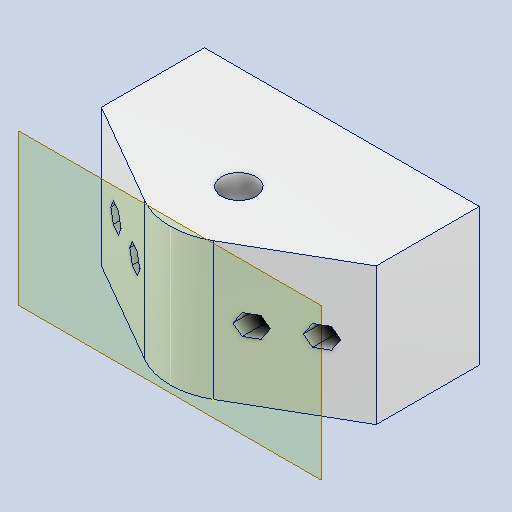
# Autodesk Inventor part: encatre sin fin
Saved by Autodesk Inventor 2023 (Build 270158000, 158)
## iProperties
Created: 2023-04-13
Part Number: encatre sin fin
Material: Aluminum 6061
Document SubType Name: Modeling
Designer: sebas
Density: 2.7 g/cm^3
Appearance: Aluminum - Flat
Author: sebas
Autodesk Inventor part; units mm, degrees
ref_plane "YZ Plane" through (0, 0, 0) normal (1, 0, 0) x (0, 1, 0)
ref_plane "XZ Plane" through (0, 0, 0) normal (0, 1, 0) x (-1, 0, 0)
ref_plane "XY Plane" through (0, 0, 0) normal (0, 0, 1) x (1, 0, 0)
sketch "Sketch1" plane through (0, 0, 0) normal (0, 1, 0) x (-1, 0, 0)
  circle A0 centre (0, 0) radius 20
  line L0 (8, 0) -> (4, -6.9282)
  line L1 (4, -6.9282) -> (-4, -6.9282)
  line L2 (-4, -6.9282) -> (-8, 0)
  line L3 (-8, 0) -> (-4, 6.9282)
  line L4 (-4, 6.9282) -> (4, 6.9282)
  line L5 (4, 6.9282) -> (8, 0)
  dimension "d1" = 40
  dimension "d5" = 8
  constraints: 12 end point, 2 coincident, 1 centre point, 13 other
  measures "d1" diameter of A0
  measures "d5" distance of A0.centre L0.start
extrude "Extrusion1" add sketch "Sketch1" along normal blind 40
sketch "Sketch2" plane through (0, 40, 0) normal (0, 1, 0) x (1, 0, 0)
  line L0 (-8, 0) -> (-4, 6.9282) projected
  line L1 (-8, 0) -> (-4, 6.9282)
  line L2 (-4, 6.9282) -> (4, 6.9282)
  line L3 (4, 6.9282) -> (8, 0)
  line L4 (8, 0) -> (4, -6.9282)
  line L5 (4, -6.9282) -> (-4, -6.9282)
  line L6 (-4, -6.9282) -> (-8, 0)
  point P0 (0, 0)
  point P1 (0, 0)
  constraints: 12 end point, 1 coincident, 13 other
extrude "Extrusion2" add sketch "Sketch2" against normal blind 10
sketch "Sketch3" plane through (0, 40, 0) normal (0, 1, 0) x (1, 0, 0)
  circle A0 centre (0, 0) radius 5
  dimension "d8" = 10
  constraints: 1 centre point, 1 coincident
  measures "d8" diameter of A0
extrude "Extrusion3" cut sketch "Sketch3" against normal blind 10
sketch "Sketch4" plane through (0, 40, 0) normal (0, 1, 0) x (1, 0, 0)
  circle A0 centre (0, 0) radius 20 projected
  line L0 (20, 0) -> (40, 0)
  line L1 (40, 0) -> (40, 20)
  line L2 (40, 20) -> (0, 20)
  line L3 (-20, 20) -> (-40, 20)
  line L4 (-40, 20) -> (-40, 0)
  line L5 (-40, 0) -> (-20, 0)
  line L6 (-20, 20) -> (0, 20)
  line L7 (-40, 0) -> (-10, -17.3205)
  line L8 (40, 0) -> (10, -17.3205)
  circle A1 centre (0, 0) radius 20
  circle A2 centre (0, 0) radius 20
  dimension "d11" = 20
  dimension "d12" = 20
  constraints: 18 end point, 5 point on circle, 4 point on line, 4 tangent, 2 centre point, 2 coincident, 2 concentric, 2 perpendicular, 1 collinear, 1 horizontal
  measures "d11" distance of L0.start L0.end
  measures "d12" distance of L3.start L3.end
extrude "Extrusion4" add sketch "Sketch4" against normal blind 40 contours L0 L8 A0 | A0 L2 L1 L0 | A0 L5 L4 L3 L6 | A0 L7 L5
sketch "Sketch5" plane through (40, 40, -20) normal (0, 0, -1) x (-1, 0, 0)
  line L0 (0, 0) -> (0, -40) projected
  line L1 (0, -20) -> (80, -20)
  line L2 (80, 0) -> (80, -40) projected
  line L3 (0, -20) -> (10, -20)
  circle A0 centre (10, -20) radius 3
  line L4 (13, -20) -> (23, -20)
  circle A1 centre (23, -20) radius 3
  line L5 (40, -40) -> (40, 0)
  circle A2 centre (70, -20) radius 3
  circle A3 centre (57, -20) radius 3
  dimension "d16" = 6
  dimension "d15" = 10
  dimension "d17" = 10
  dimension "d18" = 6
  constraints: 8 end point, 3 centre point, 2 coincident, 2 midpoint, 2 point on line, 2 symmetric about line, 1 horizontal alignment, 1 vertical, 4 other
  measures "d15" distance of L1.start L3.end
  measures "d17" distance of L4.start L4.end
  measures "d18" diameter of A1
extrude "Extrusion5" cut sketch "Sketch5" along normal mid plane 80
sketch "Sketch6" plane through (0, 40, 0) normal (0, 1, 0) x (1, 0, 0)
  line L0 (-40, 20) -> (-40, 15)
  line L1 (-40, 0) -> (-40, 20) projected
  line L2 (-40, 15) -> (44.9562, 15)
  line L3 (44.9562, 15) -> (44.9562, 24.7883)
  line L4 (44.9562, 24.7883) -> (-40, 24.7883)
  line L5 (-40, 24.7883) -> (-40, 20)
  point P0 (0, 0)
  dimension "d21" = 5
  constraints: 10 end point, 4 perpendicular, 2 point on line
  measures "d21" distance of L0.start L0.end
extrude "Extrusion6" cut sketch "Sketch6" against normal through all
sketch "Sketch7" plane through (10, 0, 17.3205) normal (0.5, 0, 0.8660254) x (0.8660254, 0, -0.5)
  point P0 (0, 0)
ref_plane "Work Plane1" through (0, 0, 20) normal (0, 0, -1) x (-1, 0, 0)
sketch "Sketch8" plane through (0, 0, 20) normal (0, 0, -1) x (-1, 0, 0)
  circle A0 centre (-30, 20) radius 3 projected
  line L0 (-28.2679, 23) -> (-26.5359, 20)
  line L1 (-26.5359, 20) -> (-28.2679, 17)
  line L2 (-28.2679, 17) -> (-31.7321, 17)
  line L3 (-31.7321, 17) -> (-33.4641, 20)
  line L4 (-33.4641, 20) -> (-31.7321, 23)
  line L5 (-31.7321, 23) -> (-28.2679, 23)
  circle A1 centre (-17, 20) radius 3 projected
  line L6 (-15.2679, 23) -> (-13.5359, 20)
  line L7 (-13.5359, 20) -> (-15.2679, 17)
  line L8 (-15.2679, 17) -> (-18.7321, 17)
  line L9 (-18.7321, 17) -> (-20.4641, 20)
  line L10 (-20.4641, 20) -> (-18.7321, 23)
  line L11 (-18.7321, 23) -> (-15.2679, 23)
  circle A2 centre (17, 20) radius 3 projected
  line L12 (18.7321, 23) -> (20.4641, 20)
  line L13 (20.4641, 20) -> (18.7321, 17)
  line L14 (18.7321, 17) -> (15.2679, 17)
  line L15 (15.2679, 17) -> (13.5359, 20)
  line L16 (13.5359, 20) -> (15.2679, 23)
  line L17 (15.2679, 23) -> (18.7321, 23)
  circle A3 centre (30, 20) radius 3 projected
  line L18 (31.7321, 23) -> (33.4641, 20)
  line L19 (33.4641, 20) -> (31.7321, 17)
  line L20 (31.7321, 17) -> (28.2679, 17)
  line L21 (28.2679, 17) -> (26.5359, 20)
  line L22 (26.5359, 20) -> (28.2679, 23)
  line L23 (28.2679, 23) -> (31.7321, 23)
  point P0 (0, 0)
  point P1 (-30, 23)
  point P2 (-17, 23)
  point P3 (17, 23)
  point P4 (30, 23)
  constraints: 48 end point, 4 coincident, 4 midpoint, 4 vertical alignment, 3 point on line, 56 other
extrude "Extrusion7" cut sketch "Sketch8" along normal blind 25
sketch "Sketch9" plane through (0, 40, 0) normal (0, 1, 0) x (1, 0, 0)
  line L0 (40, 15) -> (-40, 15) projected
  line L1 (-40, 15) -> (-40, 30)
  line L2 (-40, 0) -> (-40, 15) projected
  line L3 (-40, 30) -> (40, 30)
  line L4 (40, 15) -> (40, 0) projected
  line L5 (40, 30) -> (40, 15)
  line L6 (40, 15) -> (-40, 15)
  point P0 (0, 0)
  dimension "d26" = 15
  constraints: 8 end point, 2 collinear, 2 perpendicular
  measures "d26" distance of L0.end L1.end
extrude "Extrusion8" add sketch "Sketch9" against normal blind 40
body "Solid1"
